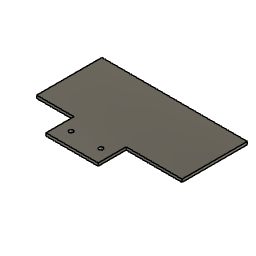
plaque (Autodesk Fusion 360 design; units mm, degrees)
Autodesk Fusion 360 part; units mm, degrees
sketch "Esquisse1" plane through (0, 0, 0) normal (0, 0, 1) x (1, 0, 0)
  line L0 (0, 0) -> (78, 0)
  line L1 (78, 0) -> (78, 50)
  line L2 (78, 50) -> (0, 50)
  line L3 (0, 50) -> (0, 0)
  line L4 (78, 0) -> (48, 0)
  line L5 (48, 0) -> (48, 15)
  line L6 (48, 15) -> (78, 15)
  line L7 (78, 15) -> (78, 0)
  circle A0 centre (42, 7.5) radius 1.1
  circle A1 centre (26, 7.5) radius 1.1
  line L8 (0, 0) -> (20, 0)
  line L9 (20, 0) -> (20, 15)
  line L10 (20, 15) -> (0, 15)
  line L11 (0, 15) -> (0, 0)
  line L12 (48, 7.5) -> (20, 7.5)
  line L13 (42, 7.5) -> (26, 7.5)
  dimension "d4" = 15
  dimension "d11" = 2.2
  dimension "d14" = 2.2
  dimension "d21" = 16
  dimension "d22" = 7.5
  dimension "d23" = 7.5
  dimension "d26" = 28
  dimension "d27" = 20
  dimension "d40" = 50
  dimension "d41" = 30
  constraint horizontal L0
  constraint vertical L1
  constraint horizontal L2
  constraint vertical L3
  constraint coincident L0.start L3.end
  constraint horizontal L4
  constraint vertical L5
  constraint horizontal L6
  constraint vertical L7
  constraint horizontal L8
  constraint vertical L9
  constraint horizontal L10
  constraint vertical L11
  constraint coincident L5 L12.start
  constraint coincident L9 L12.end
  constraint perpendicular L9 L12
  constraint coincident A0.centre L13.start
  constraint coincident A1.centre L13.end
  constraint midpoint L12 L13
  measures "d4" distance of L0.end L6.end
  measures "d11" diameter of A0
  measures "d14" diameter of A1
  measures "d21" horizontal distance of A0.centre A1.centre
  measures "d22" distance of L0 A1.centre
  measures "d23" distance of L0 A0.centre
  measures "d26" distance of L4.end L8.end
  measures "d27" distance of L3 L9
  measures "d40" distance of L0.end L1.end
  measures "d41" distance of L5.end L6.end
extrude "Extrusion3" add sketch "Esquisse1" along normal blind 1 contours A1 L12 L13 | A1 L12 L13 | A0 L12 L13 | A0 L12 L13 makes body 1 at (27.0986, 7.4452, 0.6667) makes body 2 at (42.4524, 8.5027, 0.6667)
extrude "Extrusion1" add sketch "Esquisse1" along normal blind 2 separate body contours L0 L3 L8 L9 L10 L11 | L0 L5 A0 A1 L9 L12 L13 | L1 L2 L3 L5 L6 A0 A1 L9 L10 L12 L13 | A1 L12 L13 | A1 L12 L13 | A0 L12 L13 | A0 L12 L13 makes body 3
extrude "Extrusion2" cut 1 faces at (16, 21.6667, 2) along direction (0, 0, -1) blind 1 on bodies 3 bodies 3
extrude "Extrusion4" cut 1 faces at (41.8167, 7.0732, 1) along direction (0, 0, -1) blind 1 on bodies 2 bodies 2 3
extrude "Extrusion5" cut sketch "Esquisse1" along normal blind 1 contours A1 L12 L13 | A1 L12 L13 bodies 1 3
extrude "Extrusion6" cut sketch "Esquisse1" along normal blind 1 contours L0 L3 L8 L9 L10 L11 bodies 3
extrude "Extrusion7" add 1 faces at (42, 38.3333, 1) along direction (0, 0, 1) blind 0.5 on bodies 3 bodies 3 1 2
extrude "Extrusion8" cut 1 faces at (42, 38.3333, 1.5) along direction (0, 0, -1) blind 2 on bodies 3 bodies 3
extrude "Extrusion9" add sketch "Esquisse1" along normal blind 1.5 contours L0 L5 A0 A1 L9 L12 L13 | L1 L2 L3 L5 L6 A0 A1 L9 L10 L12 L13 bodies 3
